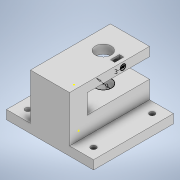
# Autodesk Inventor part: HalterungRillenKugelLager
Saved by Autodesk Inventor 2021 (Build 250183000, 183)
## iProperties
Created: 2021-03-28
Part Number: HalterungRillenKugelLager
Material: Generisch
Document SubType Name: Modeling
Designer: Elena
Density: 1 g/cm^3
Appearance: Vorgabe
Author: Elena
Autodesk Inventor part; units mm, degrees
ref_plane "YZ Plane" through (0, 0, 0) normal (1, 0, 0) x (0, 1, 0)
ref_plane "XZ Plane" through (0, 0, 0) normal (0, 1, 0) x (-1, 0, 0)
ref_plane "XY Plane" through (0, 0, 0) normal (0, 0, 1) x (1, 0, 0)
sketch "Skizze1" plane through (0, 0, 0) normal (0, 1, 0) x (-1, 0, 0)
  line L0 (0, 0) -> (17, 0)
  line L1 (17, 0) -> (17, -40)
  line L2 (17, -40) -> (0, -40)
  line L3 (0, -40) -> (0, 0)
  dimension "d0" = 17
  dimension "d1" = 40
  constraints: 8 end point, 2 parallel, 1 horizontal, 1 perpendicular
  measures "d0" distance of L1.end L2.end
  measures "d1" distance of L0.end L1.end
extrude "Extrusion1" add sketch "Skizze1" along normal blind 5
sketch "Skizze2" plane through (0, 5, 0) normal (0, 1, 0) x (1, 0, 0)
  line L0 (-17, 0) -> (0, 0) projected
  line L1 (0, 0) -> (0, 40) projected
  line L2 (-17, 0) -> (0, 0)
  line L3 (0, 0) -> (0, 10)
  line L4 (0, 10) -> (-17, 10)
  line L5 (-17, 10) -> (-17, 0)
  dimension "d4" = 10
  constraints: 8 end point, 2 parallel, 1 horizontal, 1 perpendicular, 1 point on line
  measures "d4" distance of L3.end L2.end
extrude "Extrusion2" add sketch "Skizze2" along normal blind 11
sketch "Skizze3" plane through (0, 16, 0) normal (0, 1, 0) x (1, 0, 0)
  line L0 (-17, 0) -> (0, 0) projected
  line L1 (0, 0) -> (0, 40) projected
  line L2 (-17, 0) -> (0, 0)
  line L3 (0, 0) -> (0, 40)
  line L4 (0, 40) -> (-17, 40)
  line L5 (-17, 40) -> (-17, 0)
  dimension "d7" = 17
  dimension "d8" = 40
  constraints: 8 end point, 2 parallel, 1 horizontal, 1 perpendicular
  measures "d7" distance of L4.end L1.end
  measures "d8" distance of L1.end L2.end
extrude "Extrusion3" add sketch "Skizze3" along normal blind 5
sketch "Skizze4" plane through (0, 21, 0) normal (0, 1, 0) x (1, 0, 0)
  line L0 (0, 10) -> (0, 40) projected
  line L1 (0, 40) -> (-8.5, 40)
  line L2 (-8.5, 40) -> (-8.5, 25)
  line L3 (-8.5, 25) -> (0, 25)
  line L4 (0, 25) -> (0, 40)
  circle A0 centre (-8.5, 25) radius 4.5
  point P0 (0, 0)
  dimension "d11" = 8.5
  dimension "d12" = 15
  dimension "d13" = 9
  constraints: 8 end point, 2 parallel, 1 centre point, 1 coincident, 1 horizontal, 1 perpendicular
  measures "d11" distance of L3.end L2.end
  measures "d12" distance of L2.end L1.end
  measures "d13" diameter of A0
extrude "Extrusion4" cut sketch "Skizze4" against normal blind 21 contours A0 L2 L3 | L3 L2 A0
sketch "Skizze5" plane through (0, 21, 0) normal (0, 1, 0) x (1, 0, 0)
  circle A0 centre (-8.5, 25) radius 4.5 projected
  line L0 (-8.5, 25) -> (0, 25)
  line L1 (0, 0) -> (0, 40) projected
  line L2 (0, 25) -> (-2, 25)
  line L3 (-2, 25) -> (-3.25, 25)
  line L4 (-3.25, 25) -> (-3.25, 27.55)
  line L5 (-3.25, 27.55) -> (-0.75, 27.55)
  line L6 (-0.75, 27.55) -> (-0.75, 22.45)
  line L7 (-0.75, 22.45) -> (-3.25, 22.45)
  line L8 (-3.25, 22.45) -> (-3.25, 25)
  dimension "d16" = 2
  dimension "d17" = 1.25
  dimension "d18" = 2.55
  dimension "d19" = 2.5
  dimension "d20" = 5.1
  constraints: 16 end point, 5 perpendicular, 4 point on line, 1 horizontal
  measures "d16" distance of L0.end L2.end
  measures "d17" distance of L2.end L3.end
  measures "d18" distance of L3.end L4.end
  measures "d19" distance of L4.end L5.end
  measures "d20" distance of L5.end L6.end
extrude "Extrusion5" cut sketch "Skizze5" against normal blind 5 contours L4 L5 L6 L0 | L0 L6 L7 L8
sketch "Skizze6" plane through (0, 5, 0) normal (0, 1, 0) x (1, 0, 0)
  point P0 (0, 0)
sketch "Skizze7" plane through (0, 21, 0) normal (0, 1, 0) x (1, 0, 0)
  point P0 (0, 0)
sketch "Skizze8" plane through (0, 0, 0) normal (1, 0, 0) x (0, 0, -1)
  line L0 (40, 16) -> (40, 21) projected
  line L1 (40, 20.3408) -> (25, 20.3408)
  line L2 (40, 20.3408) -> (55, 20.3408) construction
  line L3 (25, 20.3408) -> (25, 21)
  line L4 (27.55, 21) -> (22.45, 21) projected
  line L5 (25, 21) -> (25, 18.5)
  circle A0 centre (25, 18.5) radius 1.5
  point P0 (0, 0)
  dimension "d23" = 15
  dimension "d24" = 180
  dimension "d25" = 2.5
  dimension "d26" = 3
  constraints: 8 end point, 2 point on line, 1 centre point, 1 coincident, 1 collinear, 1 horizontal, 1 midpoint, 1 perpendicular
  measures "d23" distance of L1.start L1.end
  measures "d24" angle of L1 L2
  measures "d25" distance of L3.end L5.end
  measures "d26" diameter of A0
extrude "Extrusion6" cut sketch "Skizze8" against normal blind 10
sketch "Skizze9" plane through (0, 21, 0) normal (0, 1, 0) x (1, 0, 0)
  point P0 (0, 0)
sketch "Skizze10" plane through (0, 21, 0) normal (0, 1, 0) x (1, 0, 0)
  point P0 (0, 0)
sketch "Skizze11" plane through (0, 5, 0) normal (0, 1, 0) x (1, 0, 0)
  point P0 (0, 0)
sketch "Skizze12" plane through (-17, 0, -40) normal (-1, 0, 0) x (0, 0, 1)
  line L0 (40, 21) -> (0, 21) projected
  line L1 (40, 0) -> (0, 0) projected
  line L2 (40, 21) -> (30, 21)
  line L3 (30, 0) -> (40, 0)
  line L4 (40, 0) -> (40, 21)
  line L5 (30, 16) -> (0, 16) projected
  line L6 (30, 21) -> (0, 21)
  line L7 (0, 21) -> (0, 16)
  line L8 (0, 16) -> (30, 16)
  line L9 (30, 5) -> (30, 16) projected
  line L10 (30, 5) -> (0, 5)
  line L11 (0, 5) -> (0, 0)
  line L12 (0, 0) -> (30, 0)
  line L13 (30, 16) -> (30, 5)
  dimension "d29" = 10
  constraints: 20 end point, 4 equal length, 3 horizontal, 2 perpendicular, 1 point on line
  measures "d29" distance of L3.end L3.start
extrude "Extrusion7" add sketch "Skizze12" along normal blind 2.5
sketch "Skizze13" plane through (0, 0, 0) normal (1, 0, 0) x (0, 0, -1)
  line L0 (0, 0) -> (40, 0) projected
  line L1 (10, 5) -> (40, 5) projected
  line L2 (40, 0) -> (10, 0)
  line L3 (10, 5) -> (40, 5)
  line L4 (40, 5) -> (40, 0)
  line L5 (0, 0) -> (0, 21) projected
  line L6 (10, 0) -> (0, 0)
  line L7 (0, 0) -> (0, 21)
  line L8 (0, 21) -> (10, 21)
  line L9 (10, 16) -> (40, 16) projected
  line L10 (40, 16) -> (10, 16)
  line L11 (10, 21) -> (40, 21)
  line L12 (40, 21) -> (40, 16)
  line L13 (10, 5) -> (10, 16) projected
  line L14 (10, 5) -> (10, 16)
  circle A0 centre (25, 18.5) radius 1.5 projected
  circle A1 centre (25, 18.5) radius 1.5
  dimension "d32" = 3
  constraints: 20 end point, 3 horizontal, 3 parallel, 1 centre point, 1 coincident, 1 perpendicular, 1 vertical
  measures "d32" diameter of A1
extrude "Extrusion8" add sketch "Skizze13" along normal blind 2.5
sketch "Skizze14" plane through (0, 21, 0) normal (0, 1, 0) x (1, 0, 0)
  line L0 (-0.75, 27.55) -> (-3.25, 27.55) projected
  line L1 (-3.25, 22.45) -> (-3.25, 27.55) projected
  line L2 (-0.75, 27.55) -> (-3.25, 27.55)
  line L3 (-3.25, 27.55) -> (-3.25, 22.45)
  line L4 (-3.25, 22.45) -> (-0.75, 22.45)
  line L5 (-0.75, 22.45) -> (-0.75, 27.55)
  point P0 (0, 0)
  constraints: 8 end point, 2 parallel, 1 horizontal, 1 perpendicular
extrude "Extrusion9" add sketch "Skizze14" against normal blind 5
sketch "Skizze15" plane through (0, 21, 0) normal (0, 1, 0) x (1, 0, 0)
  circle A0 centre (-8.5, 25) radius 4.5 projected
  line L0 (-8.5, 25) -> (2.5, 25)
  line L1 (2.5, 26.5) -> (2.5, 23.5) projected
  line L2 (2.5, 25) -> (-4, 25)
  line L3 (2.5, 25) -> (-0.75, 25)
  line L4 (-0.75, 25) -> (-2, 25)
  line L5 (-2, 25) -> (-2, 22.45)
  line L6 (-2, 22.45) -> (0.5, 22.45)
  line L7 (0.5, 22.45) -> (0.5, 27.55)
  line L8 (0.5, 27.55) -> (-2, 27.55)
  line L9 (0.5, 27.55) -> (3, 27.55) construction
  line L10 (-2, 27.55) -> (-2, 25)
  point P0 (0, 0)
  dimension "d37" = 3.25
  dimension "d38" = 1.25
  dimension "d39" = 2.55
  dimension "d40" = 90
  dimension "d41" = 2.5
  dimension "d42" = 90
  dimension "d43" = 5.1
  dimension "d44" = 90
  dimension "d45" = 2.5
  dimension "d46" = 180
  constraints: 20 end point, 4 perpendicular, 2 midpoint, 2 point on line, 1 collinear, 1 horizontal, 1 horizontal alignment, 1 other
  measures "d37" distance of L0.end L3.end
  measures "d38" distance of L3.end L4.end
  measures "d39" distance of L4.end L5.end
  measures "d40" angle of L5 L4
  measures "d41" distance of L5.end L6.end
  measures "d42" angle of L6 L5
  measures "d43" distance of L6.end L7.end
  measures "d44" angle of L7 L6
  measures "d45" distance of L7.end L8.end
  measures "d46" angle of L8 L9
sketch "Skizze16" plane through (0, 21, 0) normal (0, 1, 0) x (1, 0, 0)
  point P0 (0, 0)
extrude "Extrusion10" cut sketch "Skizze15" against normal blind 5 contours L10 L8 L7 L0 | L0 L7 L6 L5
sketch "Skizze17" plane through (2.5, 0, 0) normal (1, 0, 0) x (0, 0, -1)
  circle A0 centre (25, 18.5) radius 1.5 projected
  circle A1 centre (25, 18.5) radius 1.5
  point P0 (0, 0)
  dimension "d49" = 3
  constraints: 1 centre point, 1 coincident
  measures "d49" diameter of A1
sketch "Skizze18" plane through (-3.25, 18.5, -25) normal (-1, 0, 0) x (0, 0, 1)
  circle A0 centre (0, 0) radius 1.5
  point P0 (25, -18.5)
  dimension "d50" = 3
  constraints: 1 centre point
  measures "d50" diameter of A0
extrude "Extrusion11" cut sketch "Skizze18" against normal blind 8
sketch "Skizze19" plane through (-19.5, 0, 0) normal (0, 0, 1) x (1, 0, 0)
  line L0 (22, 0) -> (0, 0) projected
  line L1 (0, 21) -> (0, 16) projected
  line L2 (22, 0) -> (0, 0)
  line L3 (0, 0) -> (0, 21)
  line L4 (0, 21) -> (22, 21)
  line L5 (22, 21) -> (22, 0)
  point P0 (19.5, 0)
  constraints: 8 end point, 2 parallel, 1 horizontal, 1 perpendicular
extrude "Extrusion12" add sketch "Skizze19" along normal blind 5
sketch "Skizze20" plane through (-19.5, 5, -10) normal (0, 0, -1) x (-1, 0, 0)
  line L0 (0, 11) -> (0, 0) projected
  line L1 (0, 11) -> (-22, 11) projected
  line L2 (0, 0) -> (-22, 0)
  line L3 (-22, 0) -> (-22, 11)
  line L4 (-22, 11) -> (0, 11)
  line L5 (0, 11) -> (0, 0)
  point P0 (-19.5, -5)
  constraints: 8 end point, 2 parallel, 1 horizontal, 1 perpendicular
extrude "Extrusion13" cut sketch "Skizze20" against normal blind 5
sketch "Skizze21" plane through (-19.5, 0, -40) normal (-1, 0, 0) x (0, 0, 1)
  line L0 (0, 0) -> (45, 0) projected
  line L1 (0, 5) -> (45, 5)
  line L2 (45, 5) -> (45, 0)
  line L3 (45, 0) -> (0, 0)
  line L4 (0, 0) -> (0, 5)
  point P0 (40, 0)
  constraints: 8 end point, 2 parallel, 1 horizontal, 1 perpendicular
extrude "Extrusion14" add sketch "Skizze21" along normal blind 13.5
sketch "Skizze22" plane through (2.5, 0, 0) normal (1, 0, 0) x (0, 0, -1)
  line L0 (40, 0) -> (-5, 0) projected
  line L1 (40, 5) -> (5, 5) projected
  line L2 (-5, 0) -> (40, 0)
  line L3 (40, 0) -> (40, 5)
  line L4 (40, 5) -> (-5, 5)
  line L5 (-5, 5) -> (-5, 0)
  point P0 (0, 0)
  constraints: 8 end point, 2 parallel, 1 horizontal, 1 perpendicular
extrude "Extrusion15" add sketch "Skizze22" along normal blind 13.5
sketch "Skizze23" plane through (0, 5, 0) normal (0, 1, 0) x (1, 0, 0)
  line L0 (16, 40) -> (10, 40)
  line L1 (10, 40) -> (10, 34)
  line L2 (10, 34) -> (16, 34)
  line L3 (16, 34) -> (16, 40)
  circle A0 centre (10, 34) radius 1.5
  point P0 (0, 0)
  dimension "d61" = 6
  dimension "d62" = 6
  dimension "d63" = 3
  constraints: 8 end point, 2 parallel, 1 centre point, 1 coincident, 1 horizontal, 1 perpendicular
  measures "d61" distance of L2.end L1.end
  measures "d62" distance of L1.end L0.end
  measures "d63" diameter of A0
extrude "Extrusion16" cut sketch "Skizze23" against normal blind 13.5 contours A0 L2 L1 | L1 L2 A0
sketch "Skizze24" plane through (0, 5, 0) normal (0, 1, 0) x (1, 0, 0)
  line L0 (16, -5) -> (16, 40) projected
  line L1 (16, -5) -> (10, -5)
  line L2 (10, -5) -> (10, 1)
  line L3 (10, 1) -> (16, 1)
  line L4 (16, 1) -> (16, -5)
  circle A0 centre (10, 1) radius 1.5
  point P0 (0, 0)
  dimension "d66" = 6
  dimension "d67" = 6
  dimension "d68" = 3
  constraints: 8 end point, 2 parallel, 1 centre point, 1 coincident, 1 horizontal, 1 perpendicular
  measures "d66" distance of L2.end L3.end
  measures "d67" distance of L1.end L2.end
  measures "d68" diameter of A0
extrude "Extrusion17" cut sketch "Skizze24" against normal blind 13.5 contours A0 L2 L3 | L3 L2 A0
sketch "Skizze25" plane through (0, 5, 0) normal (0, 1, 0) x (1, 0, 0)
  line L0 (-33, 40) -> (-33, -5) projected
  line L1 (-33, 40) -> (-27, 40)
  line L2 (-27, 40) -> (-27, 34)
  line L3 (-27, 34) -> (-33, 34)
  line L4 (-33, 34) -> (-33, 40)
  circle A0 centre (-27, 34) radius 1.5
  point P0 (0, 0)
  dimension "d71" = 6
  dimension "d72" = 6
  dimension "d73" = 3
  constraints: 8 end point, 2 parallel, 1 centre point, 1 coincident, 1 horizontal, 1 perpendicular
  measures "d71" distance of L2.end L3.end
  measures "d72" distance of L1.end L2.end
  measures "d73" diameter of A0
extrude "Extrusion18" cut sketch "Skizze25" against normal blind 13.5 contours A0 L2 L3 | L3 L2 A0
sketch "Skizze26" plane through (0, 5, 0) normal (0, 1, 0) x (1, 0, 0)
  line L0 (16, -5) -> (-33, -5) projected
  line L1 (-33, -5) -> (-27, -5)
  line L2 (-27, -5) -> (-27, 1)
  line L3 (-27, 1) -> (-33, 1)
  line L4 (-33, 1) -> (-33, -5)
  circle A0 centre (-27, 1) radius 1.5
  point P0 (0, 0)
  dimension "d76" = 6
  dimension "d77" = 6
  dimension "d78" = 3
  constraints: 8 end point, 2 parallel, 1 centre point, 1 coincident, 1 horizontal, 1 perpendicular
  measures "d76" distance of L3.end L2.end
  measures "d77" distance of L2.end L1.end
  measures "d78" diameter of A0
extrude "Extrusion19" cut sketch "Skizze26" against normal blind 13.5 contours A0 L3 L2 | L2 L3 A0
sketch "Skizze27" plane through (0, 5, 0) normal (0, 1, 0) x (1, 0, 0)
  line L0 (2.5, -5) -> (16, -5) projected
  line L1 (16, 40) -> (16, -5) projected
  line L2 (2.5, -5) -> (16, -5)
  line L3 (16, -5) -> (16, 40)
  line L4 (16, 40) -> (2.5, 40)
  line L5 (2.5, 40) -> (2.5, -5)
  point P0 (0, 0)
  constraints: 8 end point, 2 parallel, 1 horizontal, 1 perpendicular
extrude "Extrusion20" cut sketch "Skizze27" against normal blind 10
sketch "Skizze28" plane through (0, 5, 0) normal (0, 1, 0) x (1, 0, 0)
  line L0 (-19.5, 5) -> (-19.5, -5) projected
  line L1 (-33, -5) -> (-33, 40) projected
  line L2 (-19.5, -5) -> (-33, -5)
  line L3 (-33, -5) -> (-33, 40)
  line L4 (-33, 40) -> (-19.5, 40)
  line L5 (-19.5, 40) -> (-19.5, -5)
  point P0 (0, 0)
  constraints: 8 end point, 2 parallel, 1 horizontal, 1 perpendicular
extrude "Extrusion21" cut sketch "Skizze28" against normal blind 10
sketch "Skizze29" plane through (0, 0, 0) normal (0, -1, 0) x (1, 0, 0)
  line L0 (2.5, 5) -> (-19.5, 5) projected
  line L1 (-19.5, -40) -> (-19.5, -5) projected
  line L2 (2.5, 5) -> (-19.5, 5)
  line L3 (-19.5, 5) -> (-19.5, -40)
  line L4 (-19.5, -40) -> (2.5, -40)
  line L5 (2.5, -40) -> (2.5, 5)
  point P0 (0, 0)
  constraints: 8 end point, 2 parallel, 1 horizontal, 1 perpendicular
extrude "Extrusion22" add sketch "Skizze29" along normal blind 10
sketch "Skizze30" plane through (0, 5, 0) normal (0, 1, 0) x (1, 0, 0)
  circle A0 centre (-8.5, 25) radius 4.5 projected
  circle A1 centre (-8.5, 25) radius 4.5
  point P0 (0, 0)
  dimension "d87" = 9
  constraints: 1 centre point, 1 coincident
  measures "d87" diameter of A1
extrude "Extrusion23" add sketch "Skizze30" against normal blind 5
extrude "Extrusion24" cut sketch "Skizze30" against normal blind 15
sketch "Skizze31" plane through (2.5, 5, -40) normal (0, 0, -1) x (-1, 0, 0)
  point P0 (2.5, -5)
sketch "Skizze32" plane through (2.5, 0, 0) normal (1, 0, 0) x (0, 0, -1)
  line L0 (-5, -10) -> (-5, 21) projected
  line L1 (-5, -10) -> (40, -10)
  line L2 (40, -10) -> (40, -5)
  line L3 (40, -5) -> (-5, -5)
  line L4 (-5, -5) -> (-5, -10)
  point P0 (0, 0)
  dimension "d92" = 45
  dimension "d93" = 5
  constraints: 8 end point, 2 parallel, 1 horizontal, 1 perpendicular
  measures "d92" distance of L3.end L2.end
  measures "d93" distance of L2.end L1.end
extrude "Extrusion25" add sketch "Skizze32" along normal blind 13.5
sketch "Skizze33" plane through (-19.5, 0, -40) normal (-1, 0, 0) x (0, 0, 1)
  line L0 (45, -10) -> (0, -10) projected
  line L1 (0, -10) -> (45, -10)
  line L2 (45, -10) -> (45, -5)
  line L3 (45, -5) -> (0, -5)
  line L4 (0, -5) -> (0, -10)
  point P0 (40, 0)
  dimension "d96" = 45
  dimension "d97" = 5
  constraints: 8 end point, 2 parallel, 1 horizontal, 1 perpendicular
  measures "d96" distance of L3.end L2.end
  measures "d97" distance of L2.end L1.end
extrude "Extrusion26" add sketch "Skizze33" along normal blind 13.5
sketch "Skizze34" plane through (-19.5, -5, 5) normal (0, 1, 0) x (1, 0, 0)
  line L0 (35.5, 45) -> (-13.5, 45) projected
  line L1 (-13.5, 45) -> (-7.5, 45)
  line L2 (-7.5, 45) -> (-7.5, 39)
  line L3 (-7.5, 39) -> (-13.5, 39)
  line L4 (-13.5, 39) -> (-13.5, 45)
  circle A0 centre (-7.5, 39) radius 1.5
  point P0 (19.5, 5)
  dimension "d100" = 6
  dimension "d101" = 6
  dimension "d102" = 3
  constraints: 8 end point, 2 parallel, 1 centre point, 1 coincident, 1 horizontal, 1 perpendicular
  measures "d100" distance of L2.end L3.end
  measures "d101" distance of L1.end L2.end
  measures "d102" diameter of A0
extrude "Extrusion27" cut sketch "Skizze34" against normal blind 5 contours A0 L3 L2 | L2 L3 A0
sketch "Skizze35" plane through (-19.5, -5, 5) normal (0, 1, 0) x (1, 0, 0)
  line L0 (0, 0) -> (-13.5, 0) projected
  line L1 (-13.5, 0) -> (-7.5, 0)
  line L2 (-7.5, 0) -> (-7.5, 6)
  line L3 (-7.5, 6) -> (-13.5, 6)
  line L4 (-13.5, 6) -> (-13.5, 0)
  circle A0 centre (-7.5, 6) radius 1.5
  point P0 (19.5, 5)
  dimension "d105" = 6
  dimension "d106" = 6
  dimension "d107" = 3
  constraints: 8 end point, 2 parallel, 1 centre point, 1 coincident, 1 horizontal, 1 perpendicular
  measures "d105" distance of L3.end L2.end
  measures "d106" distance of L2.end L1.end
  measures "d107" diameter of A0
extrude "Extrusion28" cut sketch "Skizze35" against normal blind 5 contours A0 L3 L2 | L2 L3 A0
sketch "Skizze36" plane through (2.5, -5, 5) normal (0, 1, 0) x (1, 0, 0)
  line L0 (13.5, 0) -> (13.5, 45) projected
  line L1 (13.5, 45) -> (7.5, 45)
  line L2 (7.5, 45) -> (7.5, 39)
  line L3 (7.5, 39) -> (13.5, 39)
  line L4 (13.5, 39) -> (13.5, 45)
  circle A0 centre (7.5, 39) radius 1.5
  point P0 (-2.5, 5)
  dimension "d110" = 6
  dimension "d111" = 6
  dimension "d112" = 3
  constraints: 8 end point, 2 parallel, 1 centre point, 1 coincident, 1 horizontal, 1 perpendicular
  measures "d110" distance of L3.end L2.end
  measures "d111" distance of L2.end L1.end
  measures "d112" diameter of A0
sketch "Skizze37" plane through (2.5, -5, 5) normal (0, 1, 0) x (1, 0, 0)
  point P0 (-2.5, 5)
extrude "Extrusion29" cut sketch "Skizze36" against normal blind 5 contours A0 L2 L3 | L3 L2 A0
sketch "Skizze38" plane through (2.5, -5, 5) normal (0, 1, 0) x (1, 0, 0)
  line L0 (13.5, 0) -> (13.5, 45) projected
  line L1 (13.5, 0) -> (7.5, 0)
  line L2 (7.5, 0) -> (7.5, 6)
  line L3 (7.5, 6) -> (13.5, 6)
  line L4 (13.5, 6) -> (13.5, 0)
  circle A0 centre (7.5, 6) radius 1.5
  point P0 (-2.5, 5)
  dimension "d115" = 6
  dimension "d116" = 6
  dimension "d117" = 3
  constraints: 8 end point, 2 parallel, 1 centre point, 1 coincident, 1 horizontal, 1 perpendicular
  measures "d115" distance of L2.end L3.end
  measures "d116" distance of L1.end L2.end
  measures "d117" diameter of A0
extrude "Extrusion30" cut sketch "Skizze38" against normal blind 5 contours A0 L2 L3 | L3 L2 A0
